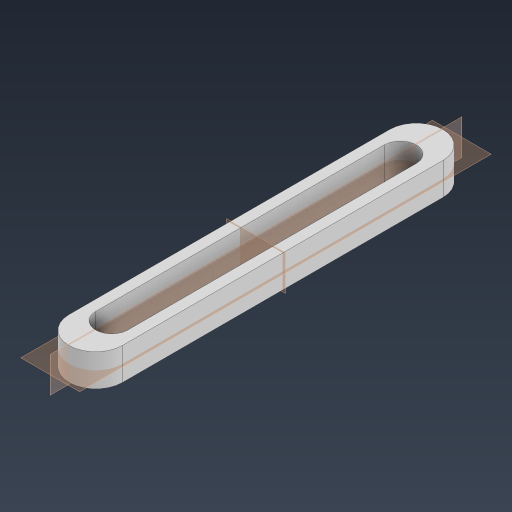
# Autodesk Inventor part: Качалка_крепления_камеры
Saved by Autodesk Inventor 2023.2 (Build 272271030, 271C)
## iProperties
Created: 2025-10-07
Part Number: Качалка_крепления_камеры
Material: Типовые
Document SubType Name: Modeling
Designer: Олег Коноваленко
Density: 1 g/cm^3
Appearance: По умолчанию
Author: Олег Коноваленко
Autodesk Inventor part; units mm, degrees
sketch "Эскиз1" plane through (0, 0, 0) normal (0, 1, 0) x (-1, 0, 0)
  line L0 (0, 15) -> (0, -15) construction
  line L1 (-2.5, 15) -> (-2.5, -15)
  line L2 (2.5, -15) -> (2.5, 15)
  arc A0 (2.5, 15) -> (-2.5, 15) centre (0, 15) ccw
  arc A1 (-2.5, -15) -> (2.5, -15) centre (0, -15) ccw
  line L3 (0, 13.5) -> (0, -13.5) construction
  line L4 (-1.5, 13.5) -> (-1.5, -13.5)
  line L5 (1.5, -13.5) -> (1.5, 13.5)
  arc A2 (1.5, 13.5) -> (-1.5, 13.5) centre (0, 13.5) ccw
  arc A3 (-1.5, -13.5) -> (1.5, -13.5) centre (0, -13.5) ccw
  line L6 (-3.5, 0) -> (3.5, 0) projected
  point P0 (0, 0)
  point P1 (0, 15)
  point P2 (-2.5, 0)
  point P3 (-1.5, 0)
  point P4 (1.5, 0)
  point P5 (2.5, 0)
  dimension "d0" = 5
  dimension "d1" = 30
  dimension "d2" = 3
  dimension "d3" = 15
  constraints: 16 end point, 9 point on circle, 8 tangent, 4 centre point, 2 midpoint, 2 parallel, 1 point on line, 1 vertical
  measures "d0" distance between parallel lines of L1 L2
  measures "d1" distance of L0.start L0.end
  measures "d2" distance between parallel lines of L4 L5
  measures "d3" distance from line of L6 point (0, 15)
extrude "Выдавливание1" add sketch "Эскиз1" along normal mid plane 3 contours A0 L2 L6 L5 A2 L4 L1 | L6 L4 A3 L5 L2 A1 L1
